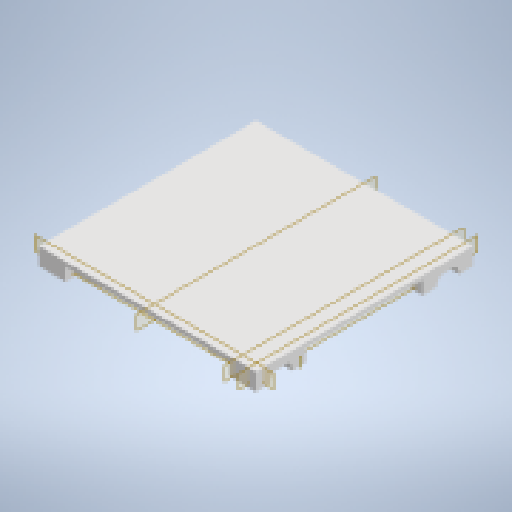
# Autodesk Inventor part: plateauV2102
Saved by Autodesk Inventor 2025.2 (Build 292293000, 293)
## iProperties
Created: 2025-02-21
Part Number: plateauV2102
Material: Générique
Document SubType Name: Modeling
Designer: antoi
Density: 1 g/cm^3
Appearance: Par défaut
Author: antoi
Autodesk Inventor part; units mm, degrees
ref_plane "YZ Plane" through (0, 0, 0) normal (1, 0, 0) x (0, 1, 0)
ref_plane "XZ Plane" through (0, 0, 0) normal (0, 1, 0) x (-1, 0, 0)
ref_plane "XY Plane" through (0, 0, 0) normal (0, 0, 1) x (1, 0, 0)
sketch "Esquisse1" plane through (0, 0, 0) normal (0, 1, 0) x (-1, 0, 0)
  line L0 (0, 0) -> (150, 0)
  line L1 (150, 0) -> (150, -150)
  line L2 (150, -150) -> (0, -150)
  line L3 (0, -150) -> (0, 0)
  dimension "d0" = 150
  dimension "d1" = 150
  constraints: 8 end point, 2 parallel, 1 horizontal, 1 perpendicular
  measures "d0" distance of L1.end L2.end
  measures "d1" distance of L0.end L1.end
extrude "Extrusion1" add sketch "Esquisse1" along normal blind 3
sketch "Esquisse2" plane through (0, 0, 0) normal (1, 0, 0) x (0, 0, -1)
  line L0 (0, 0) -> (35, 0)
  line L1 (35, 0) -> (35, -9)
  line L2 (0, -9) -> (0, 0)
  line L3 (22.4477, -3.1) -> (12.5523, -3.1)
  arc A0 (25.2, -9) -> (22.4477, -3.1) centre (17.5, -9) ccw
  arc A1 (12.5523, -3.1) -> (9.8, -9) centre (17.5, -9) ccw
  line L4 (25.2, -9) -> (35, -9)
  line L5 (9.8, -9) -> (0, -9)
  point P0 (17.4477, 0)
  point P1 (7.5523, 0)
  point P2 (5.9342, -9)
  point P3 (22.4477, 0)
  point P4 (12.5523, 0)
  dimension "d4" = 35
  dimension "d5" = 9
  constraints: 12 end point, 4 point on circle, 4 point on line, 2 centre point, 2 equal length, 2 horizontal, 1 perpendicular
  measures "d4" distance of L1.end L2.start
  measures "d5" distance of L0.end L1.end
extrude "Extrusion2" add sketch "Esquisse2" against normal blind 18.6
ref_plane "Plan de construction1" through (-150, 3, -4.9) normal (0, 0, 1) x (1, 0, 0)
ref_plane "Plan de construction2" through (0, -9, -30.1) normal (0, 0, -1) x (-1, 0, 0)
ref_plane "Plan de construction3" through (-4.5, 3, 0) normal (1, 0, 0) x (0, 0, -1)
ref_plane "Plan de construction4" through (-14.1, 3, 0) normal (1, 0, 0) x (0, 0, -1)
hole "Perçage1" at (-14.1, -9, -30.1) direction (0, 1, 0) diameter 6.3 depth 8.1
hole "Perçage2" at (-4.5, -9, -30.1) direction (0, 1, 0) diameter 6.3 depth 8.1
hole "Perçage3" at (-4.5, -9, -4.9) direction (0, 1, 0) diameter 6.3 depth 8.1
hole "Perçage4" at (-14.1, -9, -4.9) direction (0, 1, 0) diameter 6.3 depth 8.1
pattern_linear "Réseau rectangulaire1" count 2 spacing 115 along (0, 0, -1) count 2 spacing 131.4 along (-1, 0, 0) of "Extrusion2", "Perçage2", "Perçage1", "Perçage3", "Perçage4"
sketch "Esquisse5" plane through (0, 0, 0) normal (0, -1, 0) x (1, 0, 0)
  line L0 (-18.6, -5) -> (-38.6, -5)
  line L1 (-38.6, -5) -> (-38.6, -30)
  line L2 (-38.6, -30) -> (-18.6, -30)
  line L3 (-18.6, -30) -> (-18.6, -5)
  circle A0 centre (-23.1, -9.5) radius 2.3
  circle A1 centre (-23.1, -25.5) radius 2.3
  point P0 (0, 0)
  dimension "d61" = 20
  dimension "d62" = 25
  dimension "d63" = 4.6
  dimension "d64" = 4.6
  constraints: 8 end point, 2 centre point, 2 parallel, 1 horizontal, 1 perpendicular
  measures "d61" distance of L2.end L1.end
  measures "d62" distance of L1.end L0.end
  measures "d63" diameter of A0
  measures "d64" diameter of A1
extrude "Extrusion4" add sketch "Esquisse5" along normal blind 5.7
pattern_linear "Réseau rectangulaire2" count 2 spacing 115 along (0, 0, -1) of "Extrusion4"
ref_plane "Plan de construction5" through (-75, 3, 0) normal (1, 0, 0) x (0, 0, -1)
mirror "Mise en miroir1" about plane through (-75, 3, 0) normal (1, 0, 0) of "Extrusion4", "Réseau rectangulaire2"
ref_plane "Plan de construction6" through (-131.4, 0, -9.5) normal (0, 0, 1) x (1, 0, 0)
